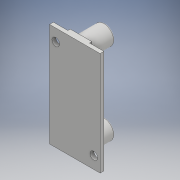
# Autodesk Inventor part: XTW-SY-8
Saved by Autodesk Inventor 2018 (Build 220112000, 112)
## iProperties
Created: 2017-10-22
Part Number: XTW-SY-8
Material: Generic
Document SubType Name: Modeling
Designer: leo2a
Density: 1 g/cm^3
Appearance: Default
Author: leo2a
Autodesk Inventor part; units mm, degrees
ref_plane "YZ Plane" through (0, 0, 0) normal (1, 0, 0) x (0, 1, 0)
ref_plane "XZ Plane" through (0, 0, 0) normal (0, 1, 0) x (-1, 0, 0)
ref_plane "XY Plane" through (0, 0, 0) normal (0, 0, 1) x (1, 0, 0)
sketch "Sketch1" plane through (0, 0, 0) normal (0, 1, 0) x (-1, 0, 0)
  line L0 (-10.5, 21.5) -> (-10.5, -21.5)
  line L1 (-10.5, -21.5) -> (10.5, -21.5)
  line L2 (10.5, -21.5) -> (10.5, 21.5)
  line L3 (10.5, 21.5) -> (-10.5, 21.5)
  line L4 (-10.5, 21.5) -> (10.5, -21.5) construction
  line L5 (-10.5, -21.5) -> (10.5, 21.5) construction
  point P0 (0, 0)
  dimension "d0" = 43
  dimension "d1" = 21
  constraints: 12 end point, 2 midpoint, 2 parallel, 1 perpendicular, 1 vertical
  measures "d0" distance of L0.start L0.end
  measures "d1" distance of L1.end L0.end
extrude "Extrusion1" add sketch "Sketch1" along normal blind 1.6
sketch "Sketch2" plane through (0, 1.6, 0) normal (0, 1, 0) x (1, 0, 0)
  line L0 (0, -21.5) -> (0, -17)
  line L1 (4.5, -12.5) -> (4.5, -21.5)
  line L2 (4.5, -21.5) -> (-4.5, -21.5)
  line L3 (-4.5, -21.5) -> (-4.5, -12.5)
  line L4 (-4.5, -12.5) -> (4.5, -12.5)
  line L5 (4.5, -12.5) -> (-4.5, -21.5) construction
  line L6 (4.5, -21.5) -> (-4.5, -12.5) construction
  line L7 (-2.2008, 0) -> (2.1177, 0)
  line L8 (4.5, 12.5) -> (4.5, 21.5)
  line L9 (4.5, 21.5) -> (-4.5, 21.5)
  line L10 (-4.5, 21.5) -> (-4.5, 12.5)
  line L11 (-4.5, 12.5) -> (4.5, 12.5)
  point P0 (0, 0)
  dimension "d4" = 4.5
  dimension "d5" = 9
  constraints: 24 end point, 4 symmetric about line, 2 midpoint, 2 parallel, 2 vertical, 1 horizontal, 1 perpendicular
  measures "d4" distance of L0.start L0.end
  measures "d5" distance of L1.end L2.end
extrude "Extrusion2" add sketch "Sketch2" along normal blind 1
sketch "Sketch3" plane through (0, 2.6, 0) normal (0, 1, 0) x (1, 0, 0)
  circle A0 centre (0, -17) radius 4
  circle A1 centre (0, 17) radius 4
  point P0 (0, 0)
  dimension "d8" = 8
  dimension "d9" = 8
  constraints: 2 centre point
  measures "d8" diameter of A0
  measures "d9" diameter of A1
extrude "Extrusion3" add sketch "Sketch3" along normal blind 10
fillet "Fillet1" radius 0.5 2 edges at (-4, 12.6, 17) (-4, 12.6, -17)
sketch "Sketch4" plane through (0, 1.6, 0) normal (0, 1, 0) x (1, 0, 0)
  line L0 (-10.5, 21.5) -> (-10.5, -21.5) projected
  line L1 (-10.5, -21.5) -> (-10.5, -16.5)
  line L2 (-10.5, -16.5) -> (-9.5, -16.5)
  line L3 (-9.5, -16.5) -> (-7.9, -16.5)
  line L4 (10.5, 21.5) -> (4.5, 21.5) projected
  line L5 (10.5, 21.5) -> (10.5, 16.5)
  line L6 (10.5, -21.5) -> (10.5, 21.5) projected
  line L7 (10.5, 16.5) -> (9.5, 16.5)
  line L8 (9.5, 16.5) -> (7.9, 16.5)
  point P0 (0, 0)
  dimension "d13" = 5
  dimension "d14" = 1
  dimension "d15" = 1.6
  dimension "d16" = 5
  dimension "d17" = 1
  dimension "d18" = 1.6
  constraints: 12 end point, 3 point on line, 2 coincident, 2 horizontal, 1 perpendicular
  measures "d13" distance of L0.end L1.end
  measures "d14" distance of L1.end L2.end
  measures "d15" distance of L2.end L3.end
  measures "d16" distance of L4.start L5.end
  measures "d17" distance of L5.end L7.end
  measures "d18" distance of L7.end L8.end
hole "Hole1" at (-7.9, 1.6, 16.5) at (7.9, 1.6, -16.5) direction (0, -1, 0) diameter 3.2 end through all clearance for "Hex Head Cap Screw ISO 24017" size "M3" standard "ISO"
body "Solid1"
